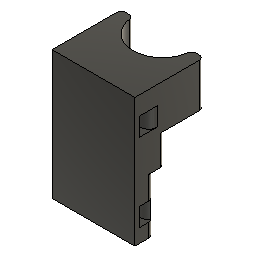
Seeed Studio Transducer Holder v4 (Autodesk Fusion 360 design; units mm, degrees)
Autodesk Fusion 360 part; units mm, degrees
sketch "Sketch1" plane through (0, 0, 0) normal (0, 0, 1) x (1, 0, 0)
  circle A0 centre (0, 0) radius 11.45
  line L0 (-6.8705, 11.9) -> (-13.7409, 0)
  line L1 (-13.7409, 0) -> (-6.8705, -11.9)
  line L2 (-6.8705, -11.9) -> (6.8705, -11.9)
  line L3 (6.8705, -11.9) -> (13.7409, 0)
  line L4 (13.7409, 0) -> (6.8705, 11.9)
  line L5 (6.8705, 11.9) -> (-6.8705, 11.9)
  line L6 (-4.6188, 8) -> (-9.2376, 0)
  line L7 (-9.2376, 0) -> (-4.6188, -8)
  line L8 (-4.6188, -8) -> (4.6188, -8)
  line L9 (4.6188, -8) -> (9.2376, 0)
  line L10 (9.2376, 0) -> (4.6188, 8)
  line L11 (4.6188, 8) -> (-4.6188, 8)
  circle A1 centre (0, 0) radius 6.375
  dimension "d2" = 22.9
  dimension "d3" = 11.9
  dimension "d15" = 8
  dimension "d24" = 12.75
  constraint coincident A0.centre A1.centre
  measures "d2" diameter of A0
  measures "d3" distance of A0.centre L5
  measures "d15" distance of A0.centre L11
  measures "d24" diameter of A1
extrude "Extrude2" add sketch "Sketch1" along normal blind 12 contours A0 | L0 L1 L2 L3 L4 L5 | L6 L7 L8 L9 L10 L11 | A1 makes body 1
extrude "Extrude3" add sketch "Sketch1" along normal blind 6.5 from surface at 12 contours A0 | L6 L7 L8 L9 L10 L11 | A1 bodies 1
extrude "Extrude4" add sketch "Sketch1" along normal blind 10 from surface at 18.5 contours A1 bodies 1
sketch "Sketch2" plane through (0, 0, 0) normal (0, 1, 0) x (1, 0, 0)
  line L0 (-9, 0) -> (9, 0)
  line L1 (9, 0) -> (9, -28)
  line L2 (9, -28) -> (-9, -28)
  line L3 (-9, -28) -> (-9, 0)
  dimension "d25" = 28
  constraint horizontal L0
  constraint vertical L1
  constraint horizontal L2
  constraint vertical L3
  constraint midpoint origin L0
  measures "d25" distance of L0.start L2.end
extrude "Extrude5" add sketch "Sketch2" against normal blind 15 separate body makes body 2
combine "Combine1" operation cut target body 2 tool bodies 1 keep tools
sketch "Sketch3" plane through (9, 0, 0) normal (1, 0, 0) x (0, 1, 0)
  line L0 (0, 28) -> (-15, 28)
  line L1 (-15, 28) -> (-15, 0)
  line L2 (-15, 0) -> (-8.2115, 0)
  line L3 (-14, 24) -> (-12, 24)
  line L4 (-12, 24) -> (-12, 20)
  line L5 (-12, 20) -> (-14, 20)
  line L6 (-14, 20) -> (-14, 24)
  line L7 (-14, 3) -> (-12, 3)
  line L8 (-12, 3) -> (-12, 7)
  line L9 (-12, 7) -> (-14, 7)
  line L10 (-14, 7) -> (-14, 3)
  line L11 (-7.0783, 12) -> (-7.0783, 18.5)
  line L12 (-8.2115, 0) -> (-8.2115, 12)
  line L13 (-8.2115, 12) -> (-7.0783, 12)
  line L14 (-7.0783, 18.5) -> (0, 18.5)
  line L15 (0, 18.5) -> (0, 28)
  constraint horizontal L3
  constraint vertical L4
  constraint horizontal L5
  constraint vertical L6
  constraint horizontal L7
  constraint vertical L8
  constraint horizontal L9
  constraint vertical L10
extrude "Extrude6" cut sketch "Sketch3" against normal blind 28 contours L3 L4 L5 L6 | L7 L8 L9 L10 bodies 2
fillet "Fillet1" radius 2 curvature continuous 4 edges at (9, -12, 22) (9, -12, 5) (-9, -12, 22) (-9, -12, 5) on bodies 2
fillet "Fillet2" radius 1 8 edges at (-9, -7.0783, 15.25) (-9, -8.2115, 6) (9, -8.2115, 6) (9, -7.0783, 15.25) (-6.375, 0, 23.25) (-9, 0, 23.25) (6.375, 0, 23.25) (9, 0, 23.25) on bodies 2
hidden bodies 1
equation "d3 = 23.8 mm / 2"
equation "d9 = 18.5 mm - 12 mm"
